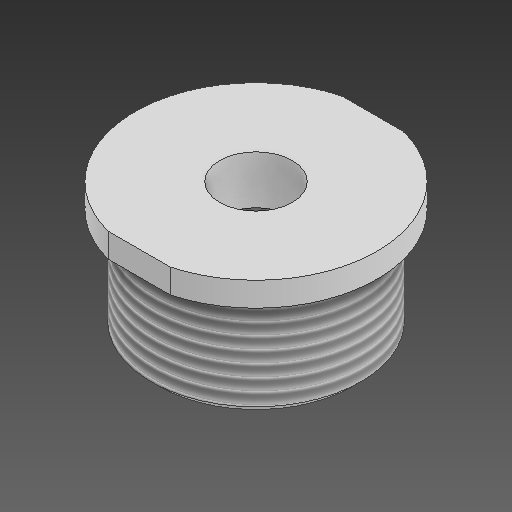
# Autodesk Inventor part: endcap
Saved by Autodesk Inventor 2021 (Build 250183000, 183)
## iProperties
Created: 2024-02-18
Part Number: endcap
Material: Generic
Document SubType Name: Modeling
Designer: top10
Density: 1 g/cm^3
Appearance: Default
Mass: 0.353429 g
Surface Area: 5.89049 cm^2
Volume: 0.353429 cm^3
Author: top10
Autodesk Inventor part; units mm, degrees
ref_plane "YZ Plane" through (0, 0, 0) normal (1, 0, 0) x (0, 1, 0)
ref_plane "XZ Plane" through (0, 0, 0) normal (0, 1, 0) x (-1, 0, 0)
ref_plane "XY Plane" through (0, 0, 0) normal (0, 0, 1) x (1, 0, 0)
sketch "Sketch1" plane through (0, 0, 0) normal (0, 0, 1) x (1, 0, 0)
  line L0 (0, 0) -> (0, -9.8072)
  line L1 (2.25, 0) -> (7.5, 0)
  line L2 (7.5, 0) -> (7.5, -1.5)
  line L3 (7.5, -1.5) -> (6.5, -1.5)
  line L4 (6.5, -1.5) -> (6.5, -8)
  line L5 (6.5, -8) -> (4, -8)
  line L6 (4, -8) -> (4, -3)
  line L7 (2.25, -1) -> (2.25, -1)
  line L8 (2.25, -1) -> (2.25, 0)
  line L9 (2.25, -1) -> (2.25, -3)
  line L10 (2.25, -3) -> (4, -3)
  dimension "d1" = 4.5
  dimension "d2" = 8
  dimension "d3" = 13
  dimension "d4" = 1.5
  dimension "d6" = 15
  dimension "d19" = 2
  dimension "d20" = 4.5
  dimension "d21" = 8
  dimension "d22" = 2.5
  dimension "d25" = 5
  dimension "d26" = 1
  constraints: 22 end point, 7 perpendicular, 3 vertical, 2 horizontal, 1 horizontal alignment
  measures "d1" diameter of L8 L0
  measures "d2" diameter of L6 L0
  measures "d3" diameter of L4 L0
  measures "d4" distance between parallel lines of L1 L3
  measures "d6" diameter of L2 L0
  measures "d19" distance between parallel lines of L7 L10
  measures "d20" diameter of L9 L0
  measures "d21" distance between parallel lines of L5 L1
  measures "d22" distance between parallel lines of L4 L6
  measures "d25" distance from line of L5.end L10
  measures "d26" distance of L7.end L1.start
revolve "Revolution1" add sketch "Sketch1" angle 360 about axis through (0, 0, 0) along (0, -1, 0)
sketch "Sketch2" plane through (0, 0, 0) normal (0, 1, 0) x (1, 0, 0)
  circle A0 centre (0, 0) radius 7.5 projected
  line L0 (-1.9203, -7.25) -> (1.9203, -7.25)
  line L1 (1.9203, -7.25) -> (1.9203, 7.25)
  line L2 (1.9203, 7.25) -> (-1.9203, 7.25)
  line L3 (-1.9203, 7.25) -> (-1.9203, -7.25)
  point P0 (0, -7.25)
  point P1 (1.9203, -7.25)
  point P2 (-1.9203, 7.25)
  point P3 (1.9203, -7.25)
  point P4 (-1.9203, 7.25)
  dimension "d29" = 14.5
  constraints: 8 end point, 2 parallel, 2 point on circle, 1 horizontal, 1 midpoint, 1 perpendicular, 1 vertical alignment
  measures "d29" distance between parallel lines of L0 L2
extrude "Extrusion1" cut sketch "Sketch2" against normal blind 10 contours L2 A0 | A0 L0
chamfer "Chamfer1" distance 0.5 angle 45 1 edges at (-6.5, -8, 0)
thread "Thread3" size "M14x0.75" class "6g" standard "ANSI Metric M Profile" full length
equation "\"d1\" = d20"
body "Solid1"
